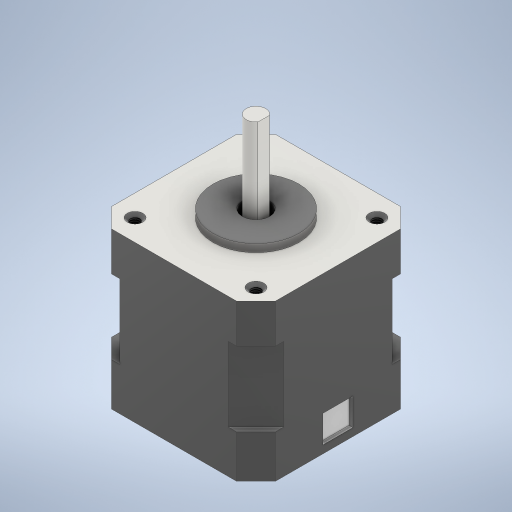
# Autodesk Inventor part: motor
Saved by Autodesk Inventor 2023 (Build 270158000, 158)
## iProperties
Created: 2023-03-04
Part Number: motor
Material: Generic
Document SubType Name: Modeling
Designer: caleb
Density: 1 g/cm^3
Appearance: Default
Author: caleb
Autodesk Inventor part; units mm, degrees
ref_plane "YZ Plane" through (0, 0, 0) normal (1, 0, 0) x (0, 1, 0)
sketch "Sketch2" plane through (0, 0, 0) normal (0, 1, 0) x (-1, 0, 0)
  line L0 (0, 0) -> (42, 0)
  line L1 (42, 0) -> (42, -42)
  line L2 (42, -42) -> (0, -42)
  line L3 (0, -42) -> (0, 0)
  circle A0 centre (21, -21) radius 11
  circle A1 centre (21, -21) radius 3.5
  circle A2 centre (21, -21) radius 2.5
  point P0 (5.5, -5.5)
  point P1 (5.5, -36.5)
  point P2 (36.5, -36.5)
  point P3 (36.5, -5.5)
  dimension "d15" = 42
  dimension "d16" = 42
  dimension "d17" = 22
  dimension "d18" = 7
  dimension "d19" = 5
  constraints: 8 end point, 3 centre point, 3 coincident, 2 parallel, 1 horizontal, 1 perpendicular
  measures "d15" distance of L1.end L2.end
  measures "d16" distance of L0.end L1.end
  measures "d17" diameter of A0
  measures "d18" diameter of A1
  measures "d19" diameter of A2
extrude "Extrusion3" add sketch "Sketch2" against normal blind 40 contours L0 L1 L2 L3 | A0
extrude "Extrusion4" add sketch "Sketch2" along normal blind 2 contours A0
hole "Hole1" at (-36.5, 0, -5.5) at (-36.5, 0, -36.5) at (-5.5, 0, -36.5) at (-5.5, 0, -5.5) direction (0, -1, 0) diameter 2.459 depth 4.5 tip angle 118 countersink diameter 4 countersink angle 90 thread size "M3x0.5" class "6H" standard "ANSI Metric M Profile"
chamfer "Chamfer1" distance 5 angle 45 4 edges at (-42, -20, 0) (0, -20, 0) (-42, -20, -42) (0, -20, -42)
ref_plane "Work Plane1" through (-5, 0, 0) normal (0.7071068, 0, 0.7071068) x (0.7071068, 0, -0.7071068)
sketch "Sketch3" plane through (-5, 0, 0) normal (0.7071068, 0, 0.7071068) x (0.7071068, 0, -0.7071068)
  line L0 (0, 0) -> (0, -40) projected
  line L1 (-22.6274, 0) -> (0, 0) projected
  line L2 (-22.6274, -40) -> (-22.6274, 0) projected
  line L3 (0, -40) -> (-22.6274, -40) projected
  line L4 (29.6985, 0) -> (29.6985, -40) projected
  line L5 (7.0711, 0) -> (29.6985, 0) projected
  line L6 (7.0711, -40) -> (7.0711, 0) projected
  line L7 (29.6985, -40) -> (7.0711, -40) projected
  line L8 (29.6985, -40) -> (29.6985, 0) projected
  line L9 (29.6985, -10) -> (28.1985, -10)
  line L10 (28.1985, -10) -> (28.1985, -29)
  line L11 (28.1985, -29) -> (29.6985, -29)
  line L12 (29.6985, -29) -> (29.6985, -10)
  line L13 (-22.6274, 0) -> (-22.6274, -40) projected
  line L14 (-22.6274, -10) -> (-21.1274, -10)
  line L15 (-21.1274, -10) -> (-21.1274, -29)
  line L16 (-21.1274, -29) -> (-22.6274, -29)
  line L17 (-22.6274, -29) -> (-22.6274, -10)
  point P0 (3.5355, 0)
  dimension "d36" = 1.5
  dimension "d50" = 1.5
  constraints: 16 end point, 4 parallel, 2 horizontal, 2 perpendicular, 2 point on line
  measures "d36" distance of L11.end L10.end
  measures "d50" distance of L15.end L16.end
extrude "Extrusion5" cut sketch "Sketch3" against normal through all contours L14 L15 L16 L2 | L4 L11 L10 L9
ref_plane "Work Plane2" through (-42, 0, -5) normal (-0.7071068, 0, 0.7071068) x (0.7071068, 0, 0.7071068)
sketch "Sketch4" plane through (-42, 0, -5) normal (-0.7071068, 0, 0.7071068) x (0.7071068, 0, 0.7071068)
  line L0 (-22.6274, -40) -> (-22.6274, 0) projected
  line L1 (0, -40) -> (-22.6274, -40) projected
  line L2 (0, 0) -> (0, -10) projected
  line L3 (-22.6274, 0) -> (0, 0) projected
  line L4 (29.6985, 0) -> (29.6985, -40) projected
  line L5 (7.0711, 0) -> (29.6985, 0) projected
  line L6 (7.0711, -40) -> (7.0711, -29) projected
  line L7 (29.6985, -40) -> (7.0711, -40) projected
  line L8 (-22.6274, -10) -> (-21.1274, -10)
  line L9 (-21.1274, -10) -> (-21.1274, -29)
  line L10 (-21.1274, -29) -> (-22.6274, -29)
  line L11 (-22.6274, -29) -> (-22.6274, -10)
  line L12 (29.6985, -40) -> (29.6985, 0) projected
  line L13 (29.6985, -10) -> (28.1985, -10)
  line L14 (28.1985, -10) -> (28.1985, -29)
  line L15 (28.1985, -29) -> (29.6985, -29)
  line L16 (29.6985, -29) -> (29.6985, -10)
  line L17 (0, -29) -> (-1.5, -29) projected
  line L18 (-1.5, -29) -> (-1.5, -10) projected
  line L19 (-1.5, -10) -> (0, -10) projected
  line L20 (0, -29) -> (0, -40) projected
  line L21 (7.0711, -10) -> (8.5711, -10) projected
  line L22 (8.5711, -10) -> (8.5711, -29) projected
  line L23 (8.5711, -29) -> (7.0711, -29) projected
  line L24 (7.0711, -10) -> (7.0711, 0) projected
  point P0 (33.234, 0)
  point P1 (29.6985, -10)
  dimension "d39" = 1.5
  dimension "d40" = 1.5
  constraints: 16 end point, 4 parallel, 4 point on line, 2 horizontal, 2 perpendicular
  measures "d39" distance of L9.end L10.end
  measures "d40" distance of L15.end L14.end
extrude "Extrusion6" cut sketch "Sketch4" against normal through all contours L0 L8 L9 L10 | L4 L15 L14 L13
extrude "Extrusion7" add sketch "Sketch2" against normal up to surface (40 mm away) contours A2
extrude "Extrusion8" add sketch "Sketch2" along normal blind 23 contours A2
sketch "Sketch5" plane through (-21, 23, -21) normal (0, 1, 0) x (1, 0, 0)
  circle A0 centre (0, 0) radius 2.5 projected
  circle A1 centre (0, 0) radius 2.5 projected
  line L0 (-2.5, 0) -> (2, 0)
  line L1 (2, 1.5) -> (2, -1.5)
  point P0 (21, -21)
  point P1 (2, -1.5)
  point P2 (2, 1.5)
  dimension "d47" = 4.5
  constraints: 4 end point, 3 point on circle, 1 horizontal, 1 vertical
  measures "d47" distance of L0.start L0.end
extrude "Extrusion9" cut sketch "Sketch5" against normal through all contours A0 L1
sketch "Sketch6" plane through (0, 0, -5) normal (1, 0, 0) x (0, 0, -1)
  line L0 (12.15, -38) -> (19.85, -38)
  line L1 (19.85, -38) -> (19.85, -31)
  line L2 (19.85, -31) -> (12.15, -31)
  line L3 (12.15, -31) -> (12.15, -38)
  point P0 (-5, 0)
  dimension "d51" = 7.7
  dimension "d52" = 7
  constraints: 8 end point, 2 parallel, 1 horizontal, 1 perpendicular
  measures "d51" distance of L2.end L1.end
  measures "d52" distance of L1.end L0.end
extrude "Extrusion10" cut sketch "Sketch6" against normal blind 1
body "Solid2"
